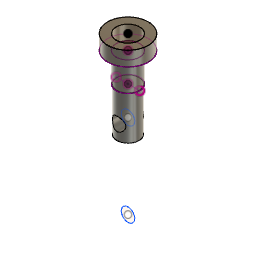
Wheel Cup (Autodesk Fusion 360 design; units mm, degrees)
Autodesk Fusion 360 part; units mm, degrees
note: some values were not read from the file. Set by a fixed rule: which sketch regions a step uses.
sketch "Sketch1" plane through (0, 0, 0) normal (0, 0, 1) x (1, 0, 0)
  circle A0 centre (0, 0) radius 7
  circle A1 centre (0, 0) radius 4
  dimension "d8" = 14
  dimension "d16" = 8
  constraint coincident A0.centre A1.centre
  constraint concentric A0 A1
  measures "d8" diameter of A0
  measures "d16" diameter of A1
extrude "Extrude2" add sketch "Sketch1" against normal blind 5 contours A0 | A1 makes body 1
extrude "Extrude1" add sketch "Sketch1" against normal blind 5 separate body contours A0 | A1 makes body 2
extrude "Extrude3" cut sketch "Sketch1" against normal blind 10 contours A1 bodies 1 2
sketch "Sketch2" plane through (0, 0, 0) normal (0, 1, 0) x (1, 0, 0)
sketch "Sketch3" plane through (0, 0, -5) normal (0, 0, -1) x (1, 0, 0)
  circle A0 centre (0, 0) radius 4.05
  circle A1 centre (0, 0) radius 4
  circle A2 centre (0, 0) radius 7
  dimension "d31" = 8.1
  constraint coincident A0.centre A1.centre
  measures "d31" diameter of A0
extrude "Extrude6" add sketch "Sketch3" along normal blind 10 contours A0 | A1 bodies 1 2
sketch "Sketch5" plane through (0, 0, 0) normal (0, 1, 0) x (1, 0, 0)
  circle A0 centre (0, 54) radius 2.3
  line L0 (4.05, 15) -> (-4.05, 15)
  circle A1 centre (0, 25) radius 2.3
  point P0 (0, 5)
  dimension "d36" = 4.6
  dimension "d40" = 4.6
  dimension "d54" = 20
  dimension "d55" = 29
  measures "d36" diameter of A0
  measures "d40" diameter of A1
  measures "d54" distance of A1.centre P0
  measures "d55" distance of A0.centre A1.centre
extrude "Extrude8" cut sketch "Sketch5" along normal mid plane 200 contours A1 bodies 1
extrude "Extrude7" cut sketch "Sketch5" along normal mid plane 200 contours A0 bodies 1
sketch "Sketch6" plane through (0, 0, -15) normal (0, 0, -1) x (1, 0, 0)
  circle A0 centre (0, 0) radius 3.8
  circle A1 centre (0, 0) radius 4.05
  dimension "d47" = 7.6
  constraint coincident A0.centre A1.centre
  measures "d47" diameter of A0
extrude "Extrude9" add sketch "Sketch6" along normal blind 15 contours A0 bodies 1
extrude "Extrude10" cut sketch "Sketch5" along normal mid plane 200 contours A1 bodies 1
extrude "Extrude11" cut sketch "Sketch5" along normal mid plane 200 contours A0 bodies 1
equation "inside_part_outer_radius = 7 mm"
equation "inside_part_inner_radius = 4 mm"
equation "inside_part_length = 5 mm"
equation "outside_part_outer_radius = 3.80 mm"
equation "outside_part_length = 15 mm"
equation "wheel_hole_distance = 29 mm"
equation "hub_nut_hole_distance = 20 mm"
equation "d8 = inside_part_outer_radius * 2"
equation "dogbone_side_gap_half_width = 2 mm"
equation "extra = 100 mm"
equation "d11 = -inside_part_length"
equation "d14 = -inside_part_length"
equation "d16 = inside_part_inner_radius * 2"
equation "d17 = -dogbone_side_gap_length"
equation "dogbone_side_gap_length = 10 mm"
equation "d31 = medium_part_outer_radius * 2"
equation "d32 = medium_part_length"
equation "dowel_pin_hole_radius = 2.3 mm"
equation "d36 = dowel_pin_hole_radius * 2"
equation "d37 = extra"
equation "d40 = dowel_pin_hole_radius * 2"
equation "d42 = extra"
equation "medium_part_outer_radius = 4.05 mm"
equation "medium_part_length = 10 mm"
equation "d47 = outside_part_outer_radius * 2"
equation "d48 = outside_part_length"
equation "d50 = extra"
equation "d52 = extra"
equation "d54 = hub_nut_hole_distance"
equation "d55 = wheel_hole_distance"
